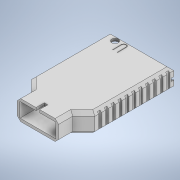
# Autodesk Inventor part: Shell
Saved by Autodesk Inventor 2021 (Build 250183000, 183)
## iProperties
Created: 2021-03-07
Part Number: Shell
Material: Generic
Document SubType Name: Modeling
Designer: mista
Density: 1 g/cm^3
Appearance: Default
Author: mista
Autodesk Inventor part; units mm, degrees
ref_plane "YZ Plane" through (0, 0, 0) normal (1, 0, 0) x (0, 1, 0)
sketch "Sketch1" plane through (0, 0, 0) normal (0, 0, 1) x (1, 0, 0)
  line L0 (0, 0) -> (33.274, 0)
  line L1 (33.274, 0) -> (33.274, 13.462)
  line L2 (33.274, 13.462) -> (0, 13.462)
  line L3 (0, 13.462) -> (0, 0)
  line L4 (-2.54, 16.002) -> (35.814, 16.002)
  line L5 (35.814, 16.002) -> (35.814, -2.54)
  line L6 (35.814, -2.54) -> (-2.54, -2.54)
  line L7 (-2.54, -2.54) -> (-2.54, 16.002)
  dimension "d0" = 33.274
  dimension "d1" = 13.462
  dimension "d2" = 2.54
  constraints: 16 end point, 4 parallel, 2 perpendicular, 1 horizontal, 3 other
  measures "d0" distance of L2.end L1.end
  measures "d1" distance of L1.end L0.end
  measures "d2" distance between parallel lines of L2 L4
sketch "Sketch1 outline for Extrusion1" plane through (0, 0, 0) normal (0, 0, 1) x (1, 0, 0)
  line L0 (-2.54, 16.002) -> (-2.54, -2.54)
  line L1 (35.814, 16.002) -> (-2.54, 16.002)
  line L2 (-2.54, -2.54) -> (35.814, -2.54)
  line L3 (35.814, -2.54) -> (35.814, 16.002)
  line L4 (0, 0) -> (0, 13.462)
  line L5 (33.274, 0) -> (0, 0)
  line L6 (33.274, 13.462) -> (33.274, 0)
  line L7 (0, 13.462) -> (33.274, 13.462)
extrude "Extrusion1" add sketch "Sketch1 outline for Extrusion1" against normal blind 13.208
sketch "Sketch3" plane through (0, 0, 0) normal (0, 0, 1) x (1, 0, 0)
  line L0 (14.986, 16.002) -> (14.986, 13.462)
  line L1 (0, 13.462) -> (33.274, 13.462)
  line L2 (35.814, 16.002) -> (-2.54, 16.002)
  line L3 (-2.54, 16.002) -> (-2.54, -2.54)
  line L4 (18.288, 16.002) -> (18.288, 13.462)
  line L5 (35.814, -2.54) -> (35.814, 16.002)
  line L6 (14.986, 16.002) -> (18.288, 16.002)
  line L7 (18.288, 13.462) -> (14.986, 13.462)
  line L8 (33.274, 13.462) -> (33.274, 0)
  line L9 (0, 0) -> (0, 13.462)
  dimension "d5" = 0
  dimension "d6" = 0
  dimension "d7" = 14.986
  dimension "d8" = 14.986
  constraints: 20 end point, 2 collinear, 1 parallel, 1 vertical
  measures "d5" distance from line of L1 L0.end
  measures "d6" distance from line of L2 L0.start
  measures "d7" distance between parallel lines of L8 L4
  measures "d8" distance between parallel lines of L0 L9
sketch "Sketch3 outline for Extrusion2" plane through (0, 0, 0) normal (0, 0, 1) x (1, 0, 0)
  line L0 (18.288, 13.462) -> (18.288, 16.002)
  line L1 (14.986, 13.462) -> (18.288, 13.462)
  line L2 (14.986, 16.002) -> (14.986, 13.462)
  line L3 (18.288, 16.002) -> (14.986, 16.002)
extrude "Extrusion2" cut sketch "Sketch3 outline for Extrusion2" against normal blind 7.62
sketch "Sketch4" plane through (0, 0, 0) normal (0, 1, 0) x (-1, 0, 0)
  line L0 (10.287, -23.368) -> (-43.561, -23.368)
  line L1 (-43.561, -23.368) -> (-43.561, -94.234)
  line L2 (-43.561, -94.234) -> (10.287, -94.234)
  line L3 (10.287, -94.234) -> (10.287, -23.368)
  circle A0 centre (-41.529, -25.4) radius 1.016
  circle A1 centre (8.255, -25.4) radius 1.016
  circle A2 centre (8.255, -92.202) radius 1.016
  circle A3 centre (-41.529, -92.202) radius 1.016
  line L4 (-33.274, -13.208) -> (0, -13.208)
  line L5 (-16.637, -13.208) -> (-16.637, -16.482475)
  circle A4 centre (-6.223, -90.17) radius 1.905
  circle A5 centre (1.905, -90.17) radius 3.302
  point P0 (0, 0)
  dimension "d11" = 53.848
  dimension "d12" = 70.866
  dimension "d14" = 2.032
  dimension "d15" = 2.032
  dimension "d16" = 2.032
  dimension "d17" = 2.032
  dimension "d18" = 2.032
  dimension "d19" = 2.032
  dimension "d20" = 2.032
  dimension "d21" = 2.032
  dimension "d22" = 2.032
  dimension "d23" = 2.032
  dimension "d24" = 2.032
  dimension "d25" = 2.032
  dimension "d26" = 26.924
  dimension "d27" = 10.16
  dimension "d69" = 16.51
  dimension "d70" = 4.064
  dimension "d71" = 3.81
  dimension "d76" = 8.382
  dimension "d77" = 4.064
  dimension "d78" = 6.604
  constraints: 10 end point, 6 centre point, 2 parallel, 1 horizontal, 1 midpoint, 1 perpendicular, 1 vertical
  measures "d11" distance of L2.end L1.end
  measures "d12" distance of L1.end L0.end
  measures "d14" diameter of A0
  measures "d15" diameter of A1
  measures "d16" diameter of A2
  measures "d17" diameter of A3
  measures "d18" distance from line of L1 A3.centre
  measures "d19" distance from line of A3.centre L2
  measures "d20" distance from line of L1 A0.centre
  measures "d21" distance from line of L0 A0.centre
  measures "d22" distance from line of L3 A1.centre
  measures "d23" distance from line of L0 A1.centre
  measures "d24" distance from line of L2 A2.centre
  measures "d25" distance from line of L3 A2.centre
  measures "d26" distance between parallel lines of L5 L3
  measures "d27" distance between parallel lines of L4 L0
  measures "d69" distance from line of L3 A4.centre
  measures "d70" distance from line of L2 A4.centre
  measures "d71" diameter of A4
  measures "d76" distance from line of L3 A5.centre
  measures "d77" distance from line of A5.centre L2
  measures "d78" diameter of A5
ref_plane "Work Plane1" through (0, 0, -23.368) normal (0, 0, -1) x (-1, 0, 0)
sketch "Sketch5" plane through (0, 0, -23.368) normal (0, 0, -1) x (-1, 0, 0)
  line L0 (10.287, 0) -> (-43.561, 0) projected
  line L1 (-43.561, 0) -> (10.287, 0)
  line L2 (10.287, 13.462) -> (10.287, 0)
  line L3 (10.287, 0) -> (-43.561, 0)
  line L4 (12.827, -2.54) -> (-46.101, -2.54)
  line L5 (-46.101, -2.54) -> (-46.101, 16.002)
  line L6 (-46.101, -2.54) -> (12.827, -2.54)
  line L7 (12.827, -2.54) -> (12.827, 16.002)
  line L8 (12.827, 16.002) -> (-46.101, 16.002)
  line L9 (-46.101, 16.002) -> (-46.101, -2.54)
  line L10 (10.287, 0) -> (-43.561, 0)
  line L11 (-43.561, 0) -> (-43.561, 13.462)
  line L12 (-43.561, 13.462) -> (10.287, 13.462)
  line L13 (10.287, 13.462) -> (10.287, 0)
  point P0 (0, 0)
  constraints: 26 end point, 4 parallel, 3 horizontal, 3 perpendicular
sketch "Sketch6" plane through (0, 0, -13.208) normal (0, 0, -1) x (-1, 0, 0)
  line L0 (-35.814, -2.54) -> (2.54, -2.54) projected
  line L1 (2.54, -2.54) -> (2.54, 16.002) projected
  line L2 (2.54, 16.002) -> (-35.814, 16.002) projected
  line L3 (-35.814, 16.002) -> (-35.814, -2.54) projected
  line L4 (0, 13.462) -> (0, 0) projected
  line L5 (0, 0) -> (-33.274, 0) projected
  line L6 (-33.274, 0) -> (-33.274, 13.462) projected
  line L7 (-33.274, 13.462) -> (0, 13.462) projected
sketch "Sketch5 outline for Extrusion3" plane through (0, 0, -23.368) normal (0, 0, -1) x (-1, 0, 0)
  line L0 (12.827, 16.002) -> (-46.101, 16.002)
  line L1 (12.827, -2.54) -> (12.827, 16.002)
  line L2 (-46.101, 16.002) -> (-46.101, -2.54)
  line L3 (-46.101, -2.54) -> (12.827, -2.54)
  line L4 (-43.561, 13.462) -> (10.287, 13.462)
  line L5 (-43.561, 0) -> (-43.561, 13.462)
  line L6 (10.287, 0) -> (-43.561, 0)
  line L7 (10.287, 13.462) -> (10.287, 0)
extrude "Extrusion3" add sketch "Sketch5 outline for Extrusion3" along normal blind 73.406
sketch "Sketch7" plane through (0, 0, -23.368) normal (0, 0, 1) x (1, 0, 0)
  line L0 (46.101, 16.002) -> (46.101, -2.54) projected
  line L1 (-12.827, 16.002) -> (46.101, 16.002) projected
  line L2 (-12.827, -2.54) -> (-12.827, 16.002) projected
  line L3 (46.101, -2.54) -> (-12.827, -2.54) projected
  line L4 (43.561, 13.462) -> (-10.287, 13.462) projected
  line L5 (43.561, 0) -> (43.561, 13.462) projected
  line L6 (-10.287, 0) -> (43.561, 0) projected
  line L7 (-10.287, 13.462) -> (-10.287, 0) projected
  point P0 (0, 0)
sketch "Sketch8" plane through (0, 0, -23.368) normal (0, 0, 1) x (1, 0, 0)
  point P0 (0, 0)
sketch "Sketch9" plane through (0, 0, 0) normal (0, 1, 0) x (-1, 0, 0)
  line L0 (2.54, -13.208) -> (-35.814, -13.208)
  line L1 (12.827, -23.368) -> (2.54, -13.208)
  line L2 (2.54, -13.208) -> (-35.814, -13.208)
  line L3 (-45.848568, -23.368) -> (12.827, -23.368)
  line L4 (-35.814, 0) -> (-35.814, -13.208)
  line L5 (-46.101, -23.368) -> (12.827, -23.368)
  line L6 (-35.814, -13.208) -> (-46.101, -23.368)
  line L7 (-46.101, -23.368) -> (12.827, -23.368)
  point P0 (0, 0)
  constraints: 10 end point, 2 collinear, 1 parallel
sketch "Sketch9 outline for Extrusion5" plane through (0, 0, 0) normal (0, 1, 0) x (-1, 0, 0)
  line L0 (12.827, -23.368) -> (2.54, -13.208)
  line L1 (-45.848568, -23.368) -> (12.827, -23.368)
  line L2 (-46.101, -23.368) -> (-45.848568, -23.368)
  line L3 (-35.814, -13.208) -> (-46.101, -23.368)
  line L4 (2.54, -13.208) -> (-35.814, -13.208)
extrude "Extrusion5" add sketch "Sketch9 outline for Extrusion5" against normal blind 2.54
sketch "Sketch11" plane through (0, 0, 0) normal (0, 1, 0) x (1, 0, 0)
  line L0 (33.274, 0) -> (0, 0)
  line L1 (33.274, 0) -> (33.274, 13.208)
  line L2 (35.814, 13.208) -> (33.274, 13.208)
  line L3 (35.814, 13.208) -> (46.101, 23.368)
  line L4 (43.561, 23.368) -> (46.101, 23.368)
  line L5 (43.561, 23.368) -> (43.561, 96.774)
  line L6 (-10.287, 96.774) -> (43.561, 96.774)
  line L7 (-10.287, 23.368) -> (-10.287, 96.774)
  line L8 (-12.827, 23.368) -> (-10.287, 23.368)
  line L9 (-12.827, 23.368) -> (-2.54, 13.208)
  line L10 (0, 13.208) -> (-2.54, 13.208)
  line L11 (0, 0) -> (0, 13.208)
  line L12 (-12.827, 23.368) -> (-2.54, 13.208)
  line L13 (-11.042139, 25.175172) -> (0, 14.269356)
  line L14 (0, 0) -> (0, 13.208)
  line L15 (0, 13.208) -> (0, 14.269356)
  line L16 (-10.287, 23.368) -> (-10.287, 96.774)
  line L17 (-10.287, 24.429356) -> (-10.287, 23.368)
  line L18 (-12.827, 23.368) -> (-10.287, 23.368)
  line L19 (-10.287, 23.368) -> (-12.827, 23.368)
  line L20 (-2.54, 0) -> (-2.54, 13.208)
  line L21 (-12.827, 23.368) -> (-2.54, 13.208)
  line L22 (-2.54, 13.208) -> (0, 13.208)
  line L23 (16.637, 13.208) -> (16.637, 17.938406)
  line L24 (46.101, 23.368) -> (43.561, 23.368)
  line L25 (46.101, 23.368) -> (35.814, 13.208)
  line L26 (44.316139, 25.175172) -> (33.274, 14.269356)
  line L27 (33.274, 13.208) -> (33.274, 14.269356)
  line L28 (43.561, 24.429356) -> (43.561, 23.368)
  line L29 (35.814, 13.208) -> (33.274, 13.208)
  point P0 (43.561, 24.429356)
  dimension "d40" = 2.54
  constraints: 26 end point, 3 point on line, 3 symmetric about line, 2 parallel, 2 vertical, 1 collinear, 1 perpendicular
  measures "d40" distance between parallel lines of L9 L13
sketch "Sketch11 outline for Extrusion7" plane through (0, 0, 0) normal (0, 1, 0) x (1, 0, 0)
  line L0 (0, 13.208) -> (0, 14.269356)
  line L1 (-2.54, 13.208) -> (0, 13.208)
  line L2 (-12.827, 23.368) -> (-2.54, 13.208)
  line L3 (-10.287, 23.368) -> (-12.827, 23.368)
  line L4 (-10.287, 24.429356) -> (-10.287, 23.368)
  line L5 (0, 14.269356) -> (-10.287, 24.429356)
  line L6 (33.274, 14.269356) -> (33.274, 13.208)
  line L7 (43.561, 24.429356) -> (33.274, 14.269356)
  line L8 (43.561, 23.368) -> (43.561, 24.429356)
  line L9 (46.101, 23.368) -> (43.561, 23.368)
  line L10 (35.814, 13.208) -> (46.101, 23.368)
  line L11 (33.274, 13.208) -> (35.814, 13.208)
extrude "Extrusion7" add sketch "Sketch11 outline for Extrusion7" along normal up to surface (13.462 mm away)
sketch "Sketch12" plane through (-12.827, 13.462, -23.368) normal (0, 1, 0) x (1, 0, 0)
  line L0 (58.928, 0) -> (55.313377, 0)
  line L1 (55.313377, 0) -> (46.101, -9.098644)
  line L2 (46.101, -9.098644) -> (46.101, -10.16)
  line L3 (48.641, -10.16) -> (46.101, -10.16)
  line L4 (48.641, -10.16) -> (58.928, 0)
  line L5 (3.614623, 0) -> (0, 0)
  line L6 (0, 0) -> (10.287, -10.16)
  line L7 (12.827, -10.16) -> (10.287, -10.16)
  line L8 (12.827, -10.16) -> (12.827, -9.098644)
  line L9 (12.827, -9.098644) -> (3.614623, 0)
  line L10 (12.827, -23.368) -> (12.827, -10.16)
  line L11 (12.827, -10.16) -> (46.101, -10.16)
  line L12 (55.313377, 0) -> (3.614623, 0)
  line L13 (55.313377, 0) -> (3.614623, 0)
  constraints: 4 end point, 1 collinear, 1 perpendicular
sketch "Sketch12 outline for Extrusion8" plane through (-12.827, 13.462, -23.368) normal (0, 1, 0) x (1, 0, 0)
  line L0 (12.827, -10.16) -> (46.101, -10.16)
  line L1 (10.287, -10.16) -> (12.827, -10.16)
  line L2 (0, 0) -> (10.287, -10.16)
  line L3 (3.614623, 0) -> (0, 0)
  line L4 (55.313377, 0) -> (3.614623, 0)
  line L5 (58.928, 0) -> (55.313377, 0)
  line L6 (48.641, -10.16) -> (58.928, 0)
  line L7 (46.101, -10.16) -> (48.641, -10.16)
extrude "Extrusion8" add sketch "Sketch12 outline for Extrusion8" along normal blind 2.54
sketch "Sketch13" plane through (0, 0, 0) normal (0, 1, 0) x (1, 0, 0)
  line L0 (43.561, 94.234) -> (-10.287, 94.234) projected
  line L1 (46.101, 96.774) -> (-12.827, 96.774) projected
  line L2 (-10.287, 94.234) -> (43.561, 94.234)
  line L3 (43.561, 94.234) -> (43.561, 96.774)
  line L4 (43.561, 96.774) -> (-10.287, 96.774)
  line L5 (-10.287, 96.774) -> (-10.287, 94.234)
  point P0 (0, 0)
  point P1 (-10.287, 96.774)
  constraints: 8 end point, 2 parallel, 1 horizontal, 1 perpendicular, 1 point on line
sketch "Sketch13 outline for Extrusion9" plane through (0, 0, 0) normal (0, 1, 0) x (1, 0, 0)
  line L0 (-10.287, 96.774) -> (-10.287, 94.234)
  line L1 (43.561, 96.774) -> (-10.287, 96.774)
  line L2 (43.561, 94.234) -> (43.561, 96.774)
  line L3 (-10.287, 94.234) -> (43.561, 94.234)
extrude "Extrusion9" add sketch "Sketch13 outline for Extrusion9" along normal up to next
chamfer "Chamfer1" distance 3.175 angle 45 14 edges at (-12.827, 16.002, -60.071) (46.101, 16.002, -60.071) (46.101, -2.54, -60.071) (-12.827, -2.54, -60.071) (16.637, 16.002, -96.774) (16.637, -2.54, -96.774) (40.9575, 16.002, -18.288) (40.9575, -2.54, -18.288) (-7.6835, 16.002, -18.288) (-7.6835, -2.54, -18.288) (35.814, 16.002, -6.604) (35.814, -2.54, -6.604) (-2.54, 16.002, -6.604) (-2.54, -2.54, -6.604)
sketch "Sketch14" plane through (14.986, 16.002, -7.62) normal (0, 1, 0) x (1, 0, 0)
  line L0 (31.115, 89.154) -> (-27.813, 89.154) projected
  line L1 (-24.638, 85.979) -> (-27.813, 89.154) projected
  line L2 (-24.638, 85.979) -> (27.94, 85.979) projected
  line L3 (31.115, 89.154) -> (27.94, 85.979) projected
  point P0 (-14.986, -7.62)
sketch "Sketch14 outline for Extrusion10" plane through (14.986, 16.002, -7.62) normal (0, 1, 0) x (1, 0, 0)
  line L0 (-24.638, 85.979) -> (27.94, 85.979)
  line L1 (-27.813, 89.154) -> (-24.638, 85.979)
  line L2 (31.115, 89.154) -> (-27.813, 89.154)
  line L3 (27.94, 85.979) -> (31.115, 89.154)
extrude "Extrusion10" cut sketch "Sketch14 outline for Extrusion10" against normal through all
sketch "Sketch16" plane through (0.635, -2.54, 0) normal (0, -1, 0) x (1, 0, 0)
  line L0 (37.211, -88.519) -> (37.211, -26.817407)
  line L1 (-5.207, -88.519) -> (37.211, -88.519)
  line L2 (-5.207, -26.817407) -> (-5.207, -88.519)
  line L3 (37.211, -26.817407) -> (-5.207, -26.817407)
  point P0 (-0.635, 0)
sketch "Sketch16 outline for Extrusion12" plane through (0.635, -2.54, 0) normal (0, -1, 0) x (1, 0, 0)
  line L0 (37.211, -88.519) -> (37.211, -26.817407)
  line L1 (-5.207, -88.519) -> (37.211, -88.519)
  line L2 (-5.207, -26.817407) -> (-5.207, -88.519)
  line L3 (37.211, -26.817407) -> (-5.207, -26.817407)
extrude "Extrusion12" cut sketch "Sketch16 outline for Extrusion12" against normal blind 0.635
sketch "Sketch4 outline for Extrusion13" plane through (0, 0, 0) normal (0, 1, 0) x (-1, 0, 0)
  circle A0 centre (-41.529, -25.4) radius 1.016
  circle A1 centre (8.255, -25.4) radius 1.016
  circle A2 centre (-41.529, -92.202) radius 1.016
  circle A3 centre (8.255, -92.202) radius 1.016
extrude "Extrusion13" add sketch "Sketch4 outline for Extrusion13" along normal blind 2.54
thicken "Thicken1" operation add thickness 0.127 both sides no extend neighbours yes toward (-0.0402659, 0, -0.999189) faces at (41.56991, 1.693333, -91.186824)
thicken "Thicken2" operation add thickness 0.127 both sides no extend neighbours yes toward (0.8451901, 0, 0.5344658) faces at (-9.113713, 1.693333, -92.745017)
thicken "Thicken3" operation add thickness 0.127 both sides no extend neighbours yes toward (0.9967573, 0, 0.0804666) faces at (-9.267705, 1.693333, -25.481754)
thicken "Thicken4" operation add thickness 0.127 both sides no extend neighbours yes toward (-0.0402659, 0, -0.999189) faces at (41.56991, 1.693333, -24.384824)
sketch "Sketch17" plane through (14.986, 16.002, -7.62) normal (0, 1, 0) x (1, 0, 0)
  arc A0 (-6.404651, 82.55) -> (-11.121349, 82.55) centre (-8.763, 82.55) ccw
  line L0 (-6.858, 82.55) -> (-6.858, 74.522669)
  line L1 (-10.668, 74.522669) -> (-10.668, 82.55)
  line L2 (-6.404651, 82.55) -> (-6.404651, 74.522669)
  line L3 (-11.121349, 74.522669) -> (-11.121349, 82.55)
  arc A1 (-6.858, 82.55) -> (-10.668, 82.55) centre (-8.763, 82.55) ccw
  line L4 (-6.404651, 74.522669) -> (-6.858, 74.522669)
  line L5 (-10.668, 74.522669) -> (-11.121349, 74.522669)
  point P0 (-14.986, -7.62)
  constraints: 12 end point, 4 point on circle, 2 centre point, 2 parallel, 2 tangent
sketch "Sketch17 outline for Extrusion14" plane through (14.986, 16.002, -7.62) normal (0, 1, 0) x (1, 0, 0)
  line L0 (-6.404651, 74.522669) -> (-6.404651, 82.55)
  line L1 (-6.858, 74.522669) -> (-6.404651, 74.522669)
  line L2 (-6.858, 82.55) -> (-6.858, 74.522669)
  arc A0 (-10.668, 82.55) -> (-6.858, 82.55) centre (-8.763, 82.55) cw
  line L3 (-10.668, 74.522669) -> (-10.668, 82.55)
  line L4 (-11.121349, 74.522669) -> (-10.668, 74.522669)
  line L5 (-11.121349, 82.55) -> (-11.121349, 74.522669)
  arc A1 (-6.404651, 82.55) -> (-11.121349, 82.55) centre (-8.763, 82.55) ccw
extrude "Extrusion14" cut sketch "Sketch17 outline for Extrusion14" against normal up to surface (2.54 mm away)
sketch "Sketch18" plane through (18.288, 13.462, 0) normal (0, -1, 0) x (1, 0, 0)
  line L0 (-10.16, -90.17) -> (-10.16, -82.142669)
  line L1 (-10.16, -82.142669) -> (-9.706651, -82.142669)
  line L2 (-9.706651, -82.142669) -> (-9.706651, -90.17)
  arc A0 (-14.423349, -90.17) -> (-9.706651, -90.17) centre (-12.065, -90.17) ccw
  line L3 (-14.423349, -90.17) -> (-14.423349, -82.142669)
  line L4 (-14.423349, -82.142669) -> (-13.97, -82.142669)
  line L5 (-13.97, -82.142669) -> (-13.97, -90.17)
  arc A1 (-13.97, -90.17) -> (-10.16, -90.17) centre (-12.065, -90.17) ccw
  line L6 (-28.575, -94.234) -> (-27.94, -93.599)
  line L7 (-27.94, -93.599) -> (24.638, -93.599)
  line L8 (24.638, -93.599) -> (25.273, -94.234)
  line L9 (25.273, -24.429356) -> (25.273, -94.234)
  line L10 (25.273, -24.429356) -> (14.986, -14.269356)
  line L11 (14.986, 0) -> (14.986, -14.269356)
  line L12 (0, 0) -> (14.986, 0)
  line L13 (0, 0) -> (0, -7.62)
  line L14 (0, -7.62) -> (-3.302, -7.62)
  line L15 (-3.302, -7.62) -> (-3.302, 0)
  line L16 (-18.288, 0) -> (-3.302, 0)
  line L17 (-18.288, 0) -> (-18.288, -14.269356)
  line L18 (-18.288, -14.269356) -> (-28.575, -24.429356)
  line L19 (-28.575, -24.429356) -> (-28.575, -94.234)
  circle A2 centre (-12.065, -90.17) radius 1.905
  point P0 (-10.16, -90.17)
  constraints: 1 centre point, 1 coincident
sketch "Sketch18 outline for Extrusion15" plane through (18.288, 13.462, 0) normal (0, -1, 0) x (1, 0, 0)
  arc A0 (-10.16, -90.17) -> (-13.97, -90.17) centre (-12.065, -90.17) ccw
  arc A1 (-13.97, -90.17) -> (-10.16, -90.17) centre (-12.065, -90.17) ccw
extrude "Extrusion15" add sketch "Sketch18 outline for Extrusion15" along normal up to surface (13.462 mm away)
sketch "Sketch4 outline for Extrusion16" plane through (0, 0, 0) normal (0, 1, 0) x (-1, 0, 0)
  circle A0 centre (1.905, -90.17) radius 3.302
extrude "Extrusion16" cut sketch "Sketch4 outline for Extrusion16" along normal through all
thicken "Thicken5" operation add thickness 0.254 both sides no extend neighbours yes toward (0.9967573, 0, -0.0804666) faces at (-5.196293, 14.308667, -89.904299)
chamfer "Chamfer2" distance 0.254 angle 45 1 edges at (1.143, 13.462, -90.17)
ref_plane "Work Plane2" through (-12.827, -2.54, -96.774) normal (0, 0, -1) x (0, 1, 0)
sketch "Sketch19" plane through (-12.827, -2.54, -96.774) normal (0, 0, -1) x (0, 1, 0)
  line L0 (0, 55.753) -> (3.175, 58.928) projected
  line L1 (2.54, 55.753) -> (0, 55.753) projected
  line L2 (2.54, 56.388) -> (2.54, 55.753) projected
  line L3 (16.002, 56.388) -> (2.54, 56.388) projected
  line L4 (16.002, 55.753) -> (16.002, 56.388) projected
  line L5 (18.542, 55.753) -> (16.002, 55.753) projected
  line L6 (15.367, 58.928) -> (18.542, 55.753) projected
  line L7 (15.367, 58.928) -> (3.175, 58.928) projected
  line L8 (3.175, 0) -> (0, 3.175) projected
  line L9 (3.175, 0) -> (15.367, 0) projected
  line L10 (18.542, 3.175) -> (15.367, 0) projected
  line L11 (18.542, 3.175) -> (16.002, 3.175) projected
  line L12 (16.002, 2.54) -> (16.002, 3.175) projected
  line L13 (2.54, 2.54) -> (16.002, 2.54) projected
  line L14 (2.54, 3.175) -> (2.54, 2.54) projected
  line L15 (2.54, 3.175) -> (0, 3.175) projected
  line L16 (2.54, 56.388) -> (16.002, 56.388) projected
  line L17 (9.271, 56.388) -> (9.271, 58.928)
  line L18 (9.271, 58.928) -> (10.541, 58.928)
  line L19 (15.367, 58.928) -> (3.175, 58.928) projected
  line L20 (10.541, 58.928) -> (8.001, 58.928)
  line L21 (8.001, 58.928) -> (8.001, 56.388)
  line L22 (8.001, 56.388) -> (10.541, 56.388)
  line L23 (10.541, 56.388) -> (10.541, 58.928)
  line L24 (16.002, 2.54) -> (2.54, 2.54) projected
  line L25 (3.175, 0) -> (15.367, 0) projected
  line L26 (10.541, 2.54) -> (8.001, 2.54)
  line L27 (8.001, 2.54) -> (8.001, 0)
  line L28 (8.001, 0) -> (10.541, 0)
  line L29 (10.541, 0) -> (10.541, 2.54)
  point P0 (2.54, 12.827)
  dimension "d86" = 1.27
  dimension "d87" = 2.54
  constraints: 20 end point, 6 point on line, 4 parallel, 2 horizontal, 2 midpoint, 2 perpendicular
  measures "d86" distance of L17.end L18.end
  measures "d87" distance of L22.end L21.end
sketch "Sketch19 outline for Extrusion17" plane through (-12.827, -2.54, -96.774) normal (0, 0, -1) x (0, 1, 0)
  line L0 (10.541, 0) -> (10.541, 2.54)
  line L1 (8.001, 0) -> (10.541, 0)
  line L2 (8.001, 2.54) -> (8.001, 0)
  line L3 (10.541, 2.54) -> (8.001, 2.54)
  line L4 (8.001, 58.928) -> (8.001, 56.388)
  line L5 (10.541, 58.928) -> (8.001, 58.928)
  line L6 (10.541, 56.388) -> (10.541, 58.928)
  line L7 (8.001, 56.388) -> (10.541, 56.388)
extrude "Extrusion17" cut sketch "Sketch19 outline for Extrusion17" against normal blind 2.54
sketch "Sketch20" plane through (14.986, 16.002, -7.62) normal (0, 1, 0) x (1, 0, 0)
  line L0 (27.94, 85.979) -> (31.115, 89.154)
  line L1 (31.115, 89.154) -> (31.115, 85.344)
  line L2 (31.115, 89.154) -> (31.115, 15.748)
  line L3 (31.115, 85.344) -> (29.845, 85.344)
  line L4 (27.94, 85.979) -> (27.94, 17.074695)
  line L5 (29.845, 85.344) -> (31.115, 85.344)
  line L6 (31.115, 85.344) -> (31.115, 82.804)
  line L7 (31.115, 82.804) -> (29.845, 82.804)
  line L8 (29.845, 82.804) -> (29.845, 85.344)
  line L9 (31.115, 76.454) -> (29.845, 76.454)
  line L10 (29.845, 76.454) -> (29.845, 78.994)
  line L11 (31.115, 78.994) -> (29.845, 78.994)
  line L12 (31.115, 78.994) -> (31.115, 76.454)
  line L13 (31.115, 70.104) -> (29.845, 70.104)
  line L14 (29.845, 70.104) -> (29.845, 72.644)
  line L15 (31.115, 72.644) -> (29.845, 72.644)
  line L16 (31.115, 72.644) -> (31.115, 70.104)
  line L17 (31.115, 63.754) -> (29.845, 63.754)
  line L18 (29.845, 63.754) -> (29.845, 66.294)
  line L19 (31.115, 66.294) -> (29.845, 66.294)
  line L20 (31.115, 66.294) -> (31.115, 63.754)
  line L21 (31.115, 57.404) -> (29.845, 57.404)
  line L22 (29.845, 57.404) -> (29.845, 59.944)
  line L23 (31.115, 59.944) -> (29.845, 59.944)
  line L24 (31.115, 59.944) -> (31.115, 57.404)
  line L25 (31.115, 51.054) -> (29.845, 51.054)
  line L26 (29.845, 51.054) -> (29.845, 53.594)
  line L27 (31.115, 53.594) -> (29.845, 53.594)
  line L28 (31.115, 53.594) -> (31.115, 51.054)
  line L29 (31.115, 44.704) -> (29.845, 44.704)
  line L30 (29.845, 44.704) -> (29.845, 47.244)
  line L31 (31.115, 47.244) -> (29.845, 47.244)
  line L32 (31.115, 47.244) -> (31.115, 44.704)
  line L33 (31.115, 38.354) -> (29.845, 38.354)
  line L34 (29.845, 38.354) -> (29.845, 40.894)
  line L35 (31.115, 40.894) -> (29.845, 40.894)
  line L36 (31.115, 40.894) -> (31.115, 38.354)
  line L37 (31.115, 32.004) -> (29.845, 32.004)
  line L38 (29.845, 32.004) -> (29.845, 34.544)
  line L39 (31.115, 34.544) -> (29.845, 34.544)
  line L40 (31.115, 34.544) -> (31.115, 32.004)
  line L41 (31.115, 25.654) -> (29.845, 25.654)
  line L42 (29.845, 25.654) -> (29.845, 28.194)
  line L43 (31.115, 28.194) -> (29.845, 28.194)
  line L44 (31.115, 28.194) -> (31.115, 25.654)
  line L45 (31.115, 19.304) -> (29.845, 19.304)
  line L46 (29.845, 19.304) -> (29.845, 21.844)
  line L47 (31.115, 21.844) -> (29.845, 21.844)
  line L48 (31.115, 21.844) -> (31.115, 19.304)
  line L49 (3.302, 0) -> (0, 0)
  line L50 (1.651, 0) -> (1.651, 2.690978)
  line L51 (-27.813, 85.344) -> (-26.543, 85.344)
  line L52 (-24.638, 85.979) -> (-24.638, 17.074695)
  line L53 (-26.543, 85.344) -> (-27.813, 85.344)
  line L54 (-27.813, 85.344) -> (-27.813, 82.804)
  line L55 (-27.813, 82.804) -> (-26.543, 82.804)
  line L56 (-26.543, 82.804) -> (-26.543, 85.344)
  line L57 (-27.813, 76.454) -> (-26.543, 76.454)
  line L58 (-26.543, 76.454) -> (-26.543, 78.994)
  line L59 (-27.813, 78.994) -> (-26.543, 78.994)
  line L60 (-27.813, 78.994) -> (-27.813, 76.454)
  line L61 (-27.813, 70.104) -> (-26.543, 70.104)
  line L62 (-26.543, 70.104) -> (-26.543, 72.644)
  line L63 (-27.813, 72.644) -> (-26.543, 72.644)
  line L64 (-27.813, 72.644) -> (-27.813, 70.104)
  line L65 (-27.813, 63.754) -> (-26.543, 63.754)
  line L66 (-26.543, 63.754) -> (-26.543, 66.294)
  line L67 (-27.813, 66.294) -> (-26.543, 66.294)
  line L68 (-27.813, 66.294) -> (-27.813, 63.754)
  line L69 (-27.813, 57.404) -> (-26.543, 57.404)
  line L70 (-26.543, 57.404) -> (-26.543, 59.944)
  line L71 (-27.813, 59.944) -> (-26.543, 59.944)
  line L72 (-27.813, 59.944) -> (-27.813, 57.404)
  line L73 (-27.813, 51.054) -> (-26.543, 51.054)
  line L74 (-26.543, 51.054) -> (-26.543, 53.594)
  line L75 (-27.813, 53.594) -> (-26.543, 53.594)
  line L76 (-27.813, 53.594) -> (-27.813, 51.054)
  line L77 (-27.813, 44.704) -> (-26.543, 44.704)
  line L78 (-26.543, 44.704) -> (-26.543, 47.244)
  line L79 (-27.813, 47.244) -> (-26.543, 47.244)
  line L80 (-27.813, 47.244) -> (-27.813, 44.704)
  line L81 (-27.813, 38.354) -> (-26.543, 38.354)
  line L82 (-26.543, 38.354) -> (-26.543, 40.894)
  line L83 (-27.813, 40.894) -> (-26.543, 40.894)
  line L84 (-27.813, 40.894) -> (-27.813, 38.354)
  line L85 (-27.813, 32.004) -> (-26.543, 32.004)
  line L86 (-26.543, 32.004) -> (-26.543, 34.544)
  line L87 (-27.813, 34.544) -> (-26.543, 34.544)
  line L88 (-27.813, 34.544) -> (-27.813, 32.004)
  line L89 (-27.813, 25.654) -> (-26.543, 25.654)
  line L90 (-26.543, 25.654) -> (-26.543, 28.194)
  line L91 (-27.813, 28.194) -> (-26.543, 28.194)
  line L92 (-27.813, 28.194) -> (-27.813, 25.654)
  line L93 (-27.813, 19.304) -> (-26.543, 19.304)
  line L94 (-26.543, 19.304) -> (-26.543, 21.844)
  line L95 (-27.813, 21.844) -> (-26.543, 21.844)
  line L96 (-27.813, 21.844) -> (-27.813, 19.304)
  point P0 (-14.986, -7.62)
  point P1 (-27.813, 34.544)
  point P2 (-27.813, 53.594)
  point P3 (-27.813, 59.944)
  point P4 (-27.813, 66.294)
  point P5 (31.115, 63.754)
  point P6 (31.115, 66.294)
  point P7 (31.115, 57.404)
  point P8 (31.115, 59.944)
  point P9 (31.115, 51.054)
  point P10 (31.115, 53.594)
  point P11 (31.115, 38.354)
  point P12 (31.115, 34.544)
  dimension "d90" = 3.81
  dimension "d91" = 1.27
  dimension "d92" = 2.54
  dimension "d95" = 6.35
  constraints: 186 end point, 57 symmetric about line, 50 vertical alignment, 22 parallel, 20 collinear, 2 perpendicular, 1 horizontal, 1 midpoint, 1 vertical, 3 other
  measures "d90" distance of L0.end L1.end
  measures "d91" distance of L1.end L3.end
  measures "d92" distance of L5.end L6.end
  measures "d95" distance of L6.end L9.start
sketch "Sketch20 outline for Extrusion18" plane through (14.986, 16.002, -7.62) normal (0, 1, 0) x (1, 0, 0)
  line L0 (-27.813, 25.654) -> (-26.543, 25.654)
  line L1 (-27.813, 28.194) -> (-27.813, 25.654)
  line L2 (-26.543, 28.194) -> (-27.813, 28.194)
  line L3 (-26.543, 25.654) -> (-26.543, 28.194)
  line L4 (-27.813, 19.304) -> (-26.543, 19.304)
  line L5 (-27.813, 21.844) -> (-27.813, 19.304)
  line L6 (-26.543, 21.844) -> (-27.813, 21.844)
  line L7 (-26.543, 19.304) -> (-26.543, 21.844)
  line L8 (-27.813, 32.004) -> (-26.543, 32.004)
  line L9 (-27.813, 34.544) -> (-27.813, 32.004)
  line L10 (-26.543, 34.544) -> (-27.813, 34.544)
  line L11 (-26.543, 32.004) -> (-26.543, 34.544)
  line L12 (-27.813, 38.354) -> (-26.543, 38.354)
  line L13 (-27.813, 40.894) -> (-27.813, 38.354)
  line L14 (-26.543, 40.894) -> (-27.813, 40.894)
  line L15 (-26.543, 38.354) -> (-26.543, 40.894)
  line L16 (-27.813, 47.244) -> (-27.813, 44.704)
  line L17 (-26.543, 47.244) -> (-27.813, 47.244)
  line L18 (-26.543, 44.704) -> (-26.543, 47.244)
  line L19 (-27.813, 44.704) -> (-26.543, 44.704)
  line L20 (-27.813, 51.054) -> (-26.543, 51.054)
  line L21 (-27.813, 53.594) -> (-27.813, 51.054)
  line L22 (-26.543, 53.594) -> (-27.813, 53.594)
  line L23 (-26.543, 51.054) -> (-26.543, 53.594)
  line L24 (-27.813, 57.404) -> (-26.543, 57.404)
  line L25 (-27.813, 59.944) -> (-27.813, 57.404)
  line L26 (-26.543, 59.944) -> (-27.813, 59.944)
  line L27 (-26.543, 57.404) -> (-26.543, 59.944)
  line L28 (-27.813, 63.754) -> (-26.543, 63.754)
  line L29 (-27.813, 66.294) -> (-27.813, 63.754)
  line L30 (-26.543, 66.294) -> (-27.813, 66.294)
  line L31 (-26.543, 63.754) -> (-26.543, 66.294)
  line L32 (-27.813, 70.104) -> (-26.543, 70.104)
  line L33 (-27.813, 72.644) -> (-27.813, 70.104)
  line L34 (-26.543, 72.644) -> (-27.813, 72.644)
  line L35 (-26.543, 70.104) -> (-26.543, 72.644)
  line L36 (-27.813, 78.994) -> (-27.813, 76.454)
  line L37 (-26.543, 78.994) -> (-27.813, 78.994)
  line L38 (-26.543, 76.454) -> (-26.543, 78.994)
  line L39 (-27.813, 76.454) -> (-26.543, 76.454)
  line L40 (-26.543, 82.804) -> (-26.543, 85.344)
  line L41 (-27.813, 82.804) -> (-26.543, 82.804)
  line L42 (-27.813, 85.344) -> (-27.813, 82.804)
  line L43 (-26.543, 85.344) -> (-27.813, 85.344)
  line L44 (29.845, 78.994) -> (29.845, 76.454)
  line L45 (31.115, 78.994) -> (29.845, 78.994)
  line L46 (31.115, 76.454) -> (31.115, 78.994)
  line L47 (29.845, 76.454) -> (31.115, 76.454)
  line L48 (29.845, 85.344) -> (29.845, 82.804)
  line L49 (31.115, 85.344) -> (29.845, 85.344)
  line L50 (31.115, 82.804) -> (31.115, 85.344)
  line L51 (29.845, 82.804) -> (31.115, 82.804)
  line L52 (29.845, 72.644) -> (29.845, 70.104)
  line L53 (31.115, 72.644) -> (29.845, 72.644)
  line L54 (31.115, 70.104) -> (31.115, 72.644)
  line L55 (29.845, 70.104) -> (31.115, 70.104)
  line L56 (29.845, 66.294) -> (29.845, 63.754)
  line L57 (31.115, 66.294) -> (29.845, 66.294)
  line L58 (31.115, 63.754) -> (31.115, 66.294)
  line L59 (29.845, 63.754) -> (31.115, 63.754)
  line L60 (29.845, 59.944) -> (29.845, 57.404)
  line L61 (31.115, 59.944) -> (29.845, 59.944)
  line L62 (31.115, 57.404) -> (31.115, 59.944)
  line L63 (29.845, 57.404) -> (31.115, 57.404)
  line L64 (29.845, 53.594) -> (29.845, 51.054)
  line L65 (31.115, 53.594) -> (29.845, 53.594)
  line L66 (31.115, 51.054) -> (31.115, 53.594)
  line L67 (29.845, 51.054) -> (31.115, 51.054)
  line L68 (29.845, 47.244) -> (29.845, 44.704)
  line L69 (31.115, 47.244) -> (29.845, 47.244)
  line L70 (31.115, 44.704) -> (31.115, 47.244)
  line L71 (29.845, 44.704) -> (31.115, 44.704)
  line L72 (29.845, 40.894) -> (29.845, 38.354)
  line L73 (31.115, 40.894) -> (29.845, 40.894)
  line L74 (31.115, 38.354) -> (31.115, 40.894)
  line L75 (29.845, 38.354) -> (31.115, 38.354)
  line L76 (29.845, 34.544) -> (29.845, 32.004)
  line L77 (31.115, 34.544) -> (29.845, 34.544)
  line L78 (31.115, 32.004) -> (31.115, 34.544)
  line L79 (29.845, 32.004) -> (31.115, 32.004)
  line L80 (29.845, 21.844) -> (29.845, 19.304)
  line L81 (31.115, 21.844) -> (29.845, 21.844)
  line L82 (31.115, 19.304) -> (31.115, 21.844)
  line L83 (29.845, 19.304) -> (31.115, 19.304)
  line L84 (29.845, 28.194) -> (29.845, 25.654)
  line L85 (31.115, 28.194) -> (29.845, 28.194)
  line L86 (31.115, 25.654) -> (31.115, 28.194)
  line L87 (29.845, 25.654) -> (31.115, 25.654)
extrude "Extrusion18" cut sketch "Sketch20 outline for Extrusion18" against normal through all
body "Solid1"
